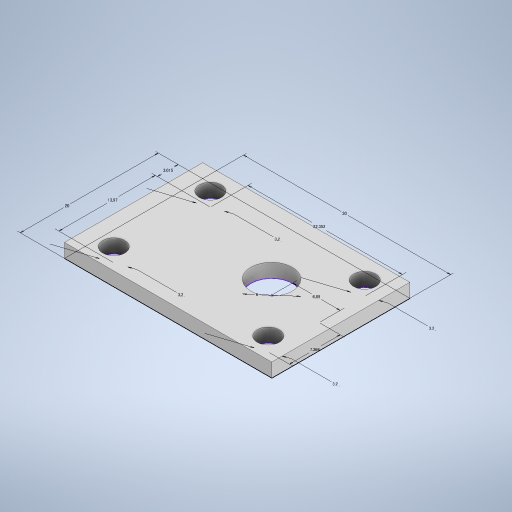
# Autodesk Inventor part: Encoder_plate1
Saved by Autodesk Inventor 2024.2 (Build 282272000, 272)
## iProperties
Created: 2024-04-17
Part Number: Encoder_plate1
Material: 一般
Document SubType Name: Modeling
Designer: towawa
Density: 1 g/cm^3
Appearance: 既定
Author: towawa
Autodesk Inventor part; units mm, degrees
ref_plane "YZ Plane" through (0, 0, 0) normal (1, 0, 0) x (0, 1, 0)
ref_plane "XZ Plane" through (0, 0, 0) normal (0, 1, 0) x (-1, 0, 0)
ref_plane "XY Plane" through (0, 0, 0) normal (0, 0, 1) x (1, 0, 0)
sketch "スケッチ1" plane through (0, 0, 0) normal (0, 1, 0) x (-1, 0, 0)
  line L0 (0, 0) -> (30, 0)
  line L1 (30, 0) -> (30, -20)
  line L2 (30, -20) -> (0, -20)
  line L3 (0, -20) -> (0, 0)
  circle A0 centre (25.889, -3.015) radius 1.6
  circle A1 centre (25.8648, -16.985) radius 1.6
  circle A2 centre (3.5128, -16.985) radius 1.6
  circle A3 centre (3.5128, -3.015) radius 1.6
  line L4 (3.5128, -3.015) -> (3.5128, -10.381)
  line L5 (3.5128, -10.381) -> (10.4023, -10.381)
  circle A4 centre (10.4023, -10.381) radius 3
  dimension "d0" = 30
  dimension "d1" = 20
  dimension "d2" = 3.2
  dimension "d3" = 3.2
  dimension "d4" = 3.2
  dimension "d5" = 3.2
  dimension "d6" = 13.97
  dimension "d7" = 3.015
  dimension "d8" = 22.352
  dimension "d14" = 7.366
  dimension "d15" = 6.8895
  dimension "d16" = 6
  constraints: 12 end point, 5 centre point, 2 parallel, 2 perpendicular, 1 coincident, 1 horizontal, 1 vertical
  measures "d0" distance of L0.start L0.end
  measures "d1" distance of L2.end L0.start
  measures "d2" diameter of A0
  measures "d3" diameter of A1
  measures "d4" diameter of A2
  measures "d5" diameter of A3
  measures "d6" distance of A0.centre A1.centre
  measures "d7" distance from line of L2 A1.centre
  measures "d8" distance of A1.centre A2.centre
  measures "d14" distance of L4.start L4.end
  measures "d15" distance of L4.end L5.end
  measures "d16" diameter of A4
extrude "押し出し1" add sketch "スケッチ1" along normal blind 2 contours L0 L1 L2 L3 | A4
extrude "押し出し2" cut sketch "スケッチ1" along normal blind 2 contours A4
